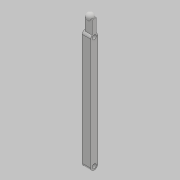
# Autodesk Inventor part: 支架3
Saved by Autodesk Inventor 2018 (Build 220112000, 112)
## iProperties
Created: 2021-03-05
Part Number: 支架3
Material: 一般
Document SubType Name: Modeling
Designer: 王鼎鈞
Density: 1 g/cm^3
Appearance: 預設
Mass: 2.43299 g
Surface Area: 19.7834 cm^2
Volume: 2.43299 cm^3
Author: 王鼎鈞
Autodesk Inventor part; units mm, degrees
sketch "草圖1" plane through (0, 0, 0) normal (1, 0, 0) x (0, 1, 0)
  line L0 (0, 0) -> (5, 0)
  line L1 (5, 0) -> (5, -85)
  line L2 (5, -85) -> (0, -85)
  line L3 (0, -85) -> (0, 0)
  dimension "d0" = 5
  dimension "d1" = 85
  constraints: 8 end point, 2 parallel, 1 horizontal, 1 perpendicular
  measures "d0" distance of L1.end L2.end
  measures "d1" distance of L0.end L1.end
extrude "擠出1" add sketch "草圖1" along normal blind 6
fillet "圓角1" radius 2.5 2 edges at (3, 5, 0) (3, 0, 0)
hole "孔1" at (6, 2.5, -2.5) direction (-1, 0, 0) diameter 3 end through all
fillet "圓角2" radius 2.5 2 edges at (3, 5, -85) (3, 0, -85)
hole "孔2" at (6, 2.5, -82.5) direction (-1, 0, 0) diameter 3 end through all
sketch "草圖2" plane through (6, 0, 0) normal (1, 0, 0) x (0, 0, -1)
  line L0 (0, -1) -> (0, 6) projected
  line L1 (0, -1) -> (0, 6) projected
  line L2 (120, 0) -> (-20, 0) projected
  circle A0 centre (82.5, 2.5) radius 1.5 projected
  circle A1 centre (2.5, 2.5) radius 1.5 projected
  arc A2 (82.5, 0) -> (82.5, 5) centre (82.5, 2.5) ccw projected
  line L3 (82.5, 5) -> (2.5, 5) projected
  arc A3 (2.5, 5) -> (2.5, 0) centre (2.5, 2.5) ccw projected
  line L4 (2.5, 0) -> (82.5, 0) projected
  circle A4 centre (98.5, 2.5) radius 1.5
  circle A5 centre (82.5, 2.5) radius 1.5 projected
  line L5 (84.5, 4) -> (98.5, 4)
  line L6 (98.5, 4) -> (98.5, 1)
  line L7 (98.5, 1) -> (84.5, 1)
  point P0 (0, 0)
  dimension "d24" = 3
  dimension "d25" = 16
  constraints: 6 end point, 2 point on circle, 1 horizontal, 1 parallel, 1 perpendicular, 1 vertical alignment, 2 other
  measures "d25" distance of A0.centre point (98.5, 2.5)
extrude "擠出2" add sketch "草圖2" against normal blind 5 contours A2 L5 A4 L7 | L6 A4 | A4 L6
ref_plane "工作平面1" through (3, 0, 0) normal (1, 0, 0) x (0, 0, -1)
sketch "草圖3" plane through (3, 0, 0) normal (1, 0, 0) x (0, 0, -1)
  arc A0 (98.5, 1) -> (98.5, 4) centre (98.5, 2.5) ccw projected
  line L0 (98.5, 1) -> (102.8586, 1)
  line L1 (102.8586, 1) -> (102.8586, 5.3685)
  line L2 (102.8586, 5.3685) -> (98.5, 5.3685)
  line L3 (98.5, 5.3685) -> (98.5, 1)
  point P0 (0, 0)
  constraints: 8 end point, 2 parallel, 1 perpendicular
extrude "擠出3" cut sketch "草圖3" along normal mid plane 6
sketch "草圖4" plane through (3, 0, 0) normal (1, 0, 0) x (0, 0, -1)
  line L0 (98.5, 4) -> (98.5, 1) projected
  arc A0 (98.5, 0) -> (98.5, 5) centre (98.5, 2.5) ccw
  line L1 (98.5, 5) -> (98.5, 0)
  point P0 (0, 0)
  dimension "d30" = 5
  constraints: 4 end point, 2 point on circle, 1 centre point, 1 midpoint, 1 vertical
  measures "d30" diameter of A0
revolve "迴轉1" add sketch "草圖4" angle 360 about axis through (3, 5, -98.5) along (0, -1, 0)
ref_plane "工作平面3" through (-79.3581, 2.5, -42.5) normal (0, 0, 1) x (1, 0, 0)
ref_plane "工作平面2" through (-79.3581, 2.5, -2.5) normal (0, 0, 1) x (1, 0, 0)
mirror "鏡射1" about plane through (-79.3581, 2.5, -42.5) normal (0, 0, 1) of "迴轉1", "擠出2", "擠出3"
sketch "草圖5" plane through (0, 0, 0) normal (-1, 0, 0) x (0, 0, 1)
  circle A0 centre (-82.5, 2.5) radius 1.5 projected
  arc A1 (-82.5, 5) -> (-82.5, 0) centre (-82.5, 2.5) ccw projected
  line L0 (-82.5, 0) -> (-2.5, 0) projected
  arc A2 (-2.5, 0) -> (-2.5, 5) centre (-2.5, 2.5) ccw projected
  line L1 (-2.5, 5) -> (-82.5, 5) projected
  circle A3 centre (-2.5, 2.5) radius 1.5 projected
  line L2 (-82.5, 0) -> (-111.7443, 0)
  line L3 (-111.7443, 0) -> (-111.7443, 9.7981)
  line L4 (-111.7443, 9.7981) -> (-82.5, 9.7981)
  line L5 (-82.5, 9.7981) -> (-82.5, 5)
  point P0 (0, 0)
  constraints: 8 end point, 2 parallel, 1 horizontal, 1 perpendicular, 1 point on circle
extrude "擠出4" cut sketch "草圖5" against normal blind 68 contours A1 L2 L3 L4 L5
sketch "草圖6" plane through (6, 0, 0) normal (1, 0, 0) x (0, 0, -1)
  line L0 (-100.5, 5.0204) -> (-0.5, 5.0204)
  line L1 (-0.5, 5.0204) -> (-0.5, -3.8226)
  line L2 (-0.5, -3.8226) -> (-100.5, -3.8226)
  line L3 (-100.5, -3.8226) -> (-100.5, 5.0204)
  circle A0 centre (2.5, 2.5) radius 1.5 projected
  point P0 (0, 0)
  dimension "d36" = 100
  dimension "d37" = 3
  constraints: 8 end point, 2 parallel, 1 horizontal, 1 perpendicular
  measures "d36" distance of L1.end L2.end
  measures "d37" distance from line of A0.centre L1
extrude "擠出5" cut sketch "草圖6" against normal blind 30.5 contours L0 L1 L2 L3
sketch "草圖7" plane through (6, 0, 0) normal (1, 0, 0) x (0, 0, -1)
  line L0 (-0.5, 4) -> (-0.5, 1) projected
  line L1 (-0.5, 4) -> (-9, 4)
  line L2 (-9, 4) -> (-9, 1)
  line L3 (-9, 1) -> (-0.5, 1)
  line L4 (-0.5, 1) -> (-0.5, 4)
  point P0 (0, 0)
  dimension "d40" = 8.5
  constraints: 8 end point, 2 parallel, 1 horizontal, 1 perpendicular
  measures "d40" distance of L3.end L2.end
extrude "擠出6" add sketch "草圖7" against normal up to surface (5 mm away)
ref_plane "工作平面5" through (3, 0, 0) normal (-1, 0, 0) x (0, 0, 1)
sketch "草圖8" plane through (3, 0, 0) normal (-1, 0, 0) x (0, 0, 1)
  line L0 (9, 4) -> (9, 1) projected
  arc A0 (9, 0) -> (9, 5) centre (9, 2.5) ccw
  line L1 (9, 5) -> (9, 0)
  point P0 (0, 0)
  dimension "d43" = 5
  constraints: 2 end point, 2 point on circle, 1 centre point, 1 midpoint, 1 vertical
  measures "d43" diameter of A0
revolve "迴轉2" add sketch "草圖8" angle 360 about axis through (3, 5, 9) along (0, -1, 0)
ref_plane "工作平面4" through (3, 0, -85) normal (-1, 0, 0) x (0, 0, 1)
